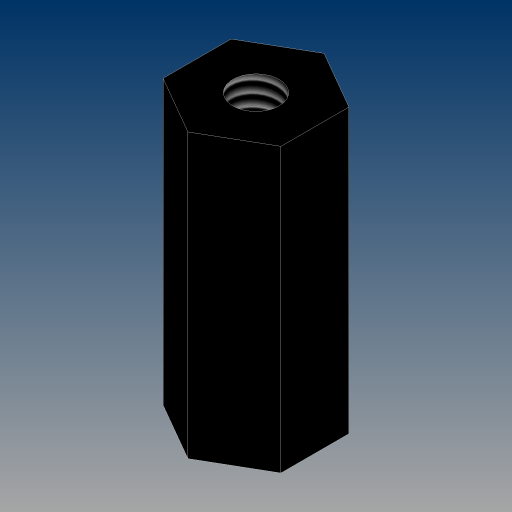
# Autodesk Inventor part: ELEV_024_SPACER1
Saved by Autodesk Inventor 2024.3 (Build 283343000, 343)
## iProperties
Created: 2024-11-28
Part Number: ELEV_024_SPACER1
Material: Aluminum 6061
Document SubType Name: Modeling
Designer: Kenji
Density: 2.7 g/cm^3
Appearance: Anodized - Black
Author: Kenji
Autodesk Inventor part; units mm, degrees
ref_plane "YZ Plane" through (0, 0, 0) normal (1, 0, 0) x (0, 1, 0)
ref_plane "XZ Plane" through (0, 0, 0) normal (0, 1, 0) x (-1, 0, 0)
ref_plane "XY Plane" through (0, 0, 0) normal (0, 0, 1) x (1, 0, 0)
sketch "Sketch1" plane through (0, 0, 0) normal (0, 1, 0) x (-1, 0, 0)
  line L0 (6.35, -3.6662) -> (0, -7.3323)
  line L1 (0, -7.3323) -> (-6.35, -3.6662)
  line L2 (-6.35, -3.6662) -> (-6.35, 3.6662)
  line L3 (-6.35, 3.6662) -> (0, 7.3323)
  line L4 (0, 7.3323) -> (6.35, 3.6662)
  line L5 (6.35, 3.6662) -> (6.35, -3.6662)
  point P0 (0, 0)
  point P1 (0, 0)
  point P2 (0, 0)
  dimension "d0" = 12.7
  constraints: 12 end point, 2 coincident, 1 vertical, 13 other
  measures "d0" distance between parallel lines of L2 L5
extrude "Extrusion1" add sketch "Sketch1" along normal blind 30.48
hole "Hole1" at (0, 0, 0) direction (0, 1, 0) diameter 4.9784 end through all thread size "1/4-20 UNC" class "2B" standard "ANSI Unified Screw Threads"
body "Solid1"
